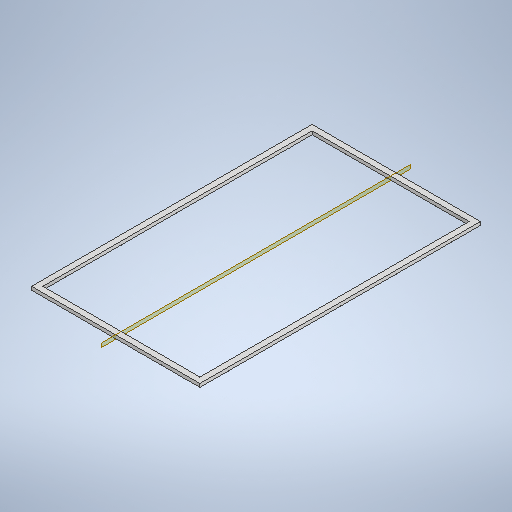
# Autodesk Inventor part: medidor
Saved by Autodesk Inventor 2025.1 (Build 291241020, 241B)
## iProperties
Created: 2024-11-27
Part Number: medidor
Material: Genérico
Document SubType Name: Modeling
Designer: ctamashiro
Density: 1 g/cm^3
Appearance: Valor por defecto
Author: ctamashiro
Autodesk Inventor part; units mm, degrees
ref_plane "YZ Plane" through (0, 0, 0) normal (1, 0, 0) x (0, 1, 0)
ref_plane "XZ Plane" through (0, 0, 0) normal (0, 1, 0) x (-1, 0, 0)
ref_plane "XY Plane" through (0, 0, 0) normal (0, 0, 1) x (1, 0, 0)
sketch "Boceto1" plane through (0, 0, 0) normal (0, 1, 0) x (-1, 0, 0)
  line L0 (-75, -125) -> (75, -125)
  line L1 (75, -125) -> (75, 125)
  line L2 (75, 125) -> (-75, 125)
  line L3 (-75, 125) -> (-75, -125)
  line L4 (-75, -125) -> (75, 125) construction
  line L5 (75, -125) -> (-75, 125) construction
  line L6 (70, 120) -> (70, -120)
  line L7 (70, -120) -> (-70, -120)
  line L8 (-70, -120) -> (-70, 120)
  line L9 (-70, 120) -> (70, 120)
  line L10 (-75, 125) -> (-75, 100)
  line L11 (-75, 100) -> (-70, 100) construction
  line L12 (-75, 100) -> (-75, 50)
  line L13 (-75, 50) -> (-70, 50) construction
  line L14 (-75, 50) -> (-75, 0)
  line L15 (-75, 100.5) -> (-70, 100.5)
  line L16 (-70, 100.5) -> (-70, 99.5)
  line L17 (-70, 99.5) -> (-75, 99.5)
  line L18 (-75, 99.5) -> (-75, 100.5)
  line L19 (-75, 100.5) -> (-70, 99.5) construction
  line L20 (-70, 100.5) -> (-75, 99.5) construction
  line L21 (-75, 49.5) -> (-70, 49.5)
  line L22 (-70, 49.5) -> (-70, 50.5)
  line L23 (-70, 50.5) -> (-75, 50.5)
  line L24 (-75, 50.5) -> (-75, 49.5)
  line L25 (-75, 49.5) -> (-70, 50.5) construction
  line L26 (-70, 49.5) -> (-75, 50.5) construction
  line L27 (0, 125) -> (-20, 125) construction
  line L28 (-20, 125) -> (-40, 125) construction
  line L29 (-40, 125) -> (-60, 125) construction
  line L30 (-20, 125) -> (-20, 120) construction
  line L31 (-40, 125) -> (-40, 120) construction
  line L32 (-60, 125) -> (-60, 120) construction
  line L33 (-20.5, 120) -> (-19.5, 120)
  line L34 (-19.5, 120) -> (-19.5, 125)
  line L35 (-19.5, 125) -> (-20.5, 125)
  line L36 (-20.5, 125) -> (-20.5, 120)
  line L37 (-20.5, 120) -> (-19.5, 125) construction
  line L38 (-19.5, 120) -> (-20.5, 125) construction
  line L39 (-40.5, 120) -> (-39.5, 120)
  line L40 (-39.5, 120) -> (-39.5, 125)
  line L41 (-39.5, 125) -> (-40.5, 125)
  line L42 (-40.5, 125) -> (-40.5, 120)
  line L43 (-40.5, 120) -> (-39.5, 125) construction
  line L44 (-39.5, 120) -> (-40.5, 125) construction
  line L45 (-60.5, 120) -> (-59.5, 120)
  line L46 (-59.5, 120) -> (-59.5, 125)
  line L47 (-59.5, 125) -> (-60.5, 125)
  line L48 (-60.5, 125) -> (-60.5, 120)
  line L49 (-60.5, 120) -> (-59.5, 125) construction
  line L50 (-59.5, 120) -> (-60.5, 125) construction
  line L51 (0, 125) -> (0, 120) construction
  line L52 (-0.5, 120) -> (0.5, 120)
  line L53 (0.5, 120) -> (0.5, 125)
  line L54 (0.5, 125) -> (-0.5, 125)
  line L55 (-0.5, 125) -> (-0.5, 120)
  line L56 (-0.5, 120) -> (0.5, 125) construction
  line L57 (0.5, 120) -> (-0.5, 125) construction
  line L58 (-70, 0) -> (-75, 0) construction
  line L59 (-75, -0.5) -> (-70, -0.5)
  line L60 (-70, -0.5) -> (-70, 0.5)
  line L61 (-70, 0.5) -> (-75, 0.5)
  line L62 (-75, 0.5) -> (-75, -0.5)
  line L63 (-75, -0.5) -> (-70, 0.5) construction
  line L64 (-70, -0.5) -> (-75, 0.5) construction
  point P0 (0, 0)
  point P1 (-72.5, 100)
  point P2 (-72.5, 50)
  point P3 (-20, 122.5)
  point P4 (-40, 122.5)
  point P5 (-60, 122.5)
  point P6 (0, 122.5)
  point P7 (-72.5, 0)
  point P8 (-75, 0.5)
  point P9 (-75, -0.5)
  point P10 (-70, -0.5)
  point P11 (-75, 50.5)
  point P12 (-75, 49.5)
  point P13 (-70, 100.5)
  point P14 (-0.5, 125)
  point P15 (-0.5, 120)
  point P16 (0.5, 120)
  point P17 (0.5, 125)
  point P18 (-20.5, 125)
  point P19 (-19.5, 125)
  point P20 (-40.5, 125)
  point P21 (-40.5, 120)
  point P22 (-39.5, 120)
  point P23 (-39.5, 125)
  point P24 (-60.5, 120)
  point P25 (-59.5, 120)
  point P26 (-59.5, 125)
  dimension "d0" = 150
  dimension "d1" = 250
  dimension "d2" = 5
  dimension "d5" = 25
  dimension "d6" = 50
  dimension "d7" = 50
  dimension "d8" = 1
  dimension "d9" = 1
  dimension "d10" = 20
  dimension "d11" = 20
  dimension "d12" = 20
  dimension "d13" = 1
  dimension "d14" = 1
  dimension "d15" = 1
  dimension "d16" = 1
  dimension "d17" = 1
  constraints: 130 end point, 27 midpoint, 18 parallel, 17 point on line, 14 perpendicular, 8 horizontal, 3 other
  measures "d0" distance of L2.end L1.end
  measures "d1" distance of L1.end L0.end
  measures "d2" distance between parallel lines of L1 L6
  measures "d5" distance of L2.end L10.end
  measures "d6" distance of L10.end L12.end
  measures "d7" distance of L12.end L14.end
  measures "d8" distance of L15.end L16.end
  measures "d9" distance of L22.end L21.end
  measures "d10" distance of L27.start L27.end
  measures "d11" distance of L27.end L28.end
  measures "d12" distance of L28.end L29.end
  measures "d13" distance of L35.end L34.end
  measures "d14" distance of L41.end L40.end
  measures "d15" distance of L47.end L46.end
  measures "d16" distance of L54.end L53.end
  measures "d17" distance of L60.end L59.end
extrude "Extrusión1" add sketch "Boceto1" along normal blind 3 contours L3 L59 L8 L7 L6 L9 L53 L2 L1 L0 | L3 L61 L8 L59 | L53 L9 L55 L2 | L3 L21 L8 L61 | L55 L9 L34 L2 | L3 L23 L8 L21 | L34 L9 L36 L2 | L23 L3 L17 L8 | L36 L9 L40 L2 | L17 L3 L15 L8 | L40 L9 L42 L2 | L15 L3 L2 L48 L9 L8 | L42 L9 L46 L2 | L46 L9 L48 L2
extrude "Extrusión2" add sketch "Boceto1" against normal blind 0.2 contours L3 L61 L8 L59 | L53 L9 L55 L2 | L3 L23 L8 L21 | L34 L9 L36 L2 | L17 L3 L15 L8 | L40 L9 L42 L2 | L46 L9 L48 L2
mirror "Simetría1" about plane through (0, 0, 0) normal (1, 0, 0) of "Extrusión2", "Extrusión1"
mirror "Simetría2" about plane through (0, 0, 0) normal (0, 0, 1) of "Extrusión2", "Extrusión1", "Simetría1"
ref_plane "Plano de trabajo1" through (0, 0, 0) normal (1, 0, 0) x (0, 1, 0)
ref_plane "Plano de trabajo2" through (0, 0, 0) normal (-1, 0, 0) x (0, 1, 0)
ref_plane "Plano de trabajo3" through (0, 0, 0) normal (-1, 0, 0) x (0, 1, 0)
